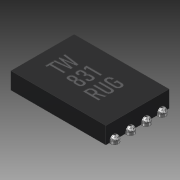
# Autodesk Inventor part: ATECC608A No Lead Crypto Auth
Saved by Autodesk Inventor 2016 (Build 200138000, 138)
## iProperties
Created: 2019-08-17
Part Number: ATECC608A No Lead Crypto Auth
Material: Generic
Document SubType Name: Modeling
Designer: Orest
Mass: 0.00326775 g
Surface Area: 0.184366 cm^2
Volume: 0.00326775 cm^3
Density: 1 g/cm^3
Appearance: Smooth - Black (BGA)
Catalog Web Link: http://ww1.microchip.com/downloads/en/DeviceDoc/40001977A.pdf
Author: Orest
Autodesk Inventor part; units mm, degrees
ref_plane "YZ Plane" through (0, 0, 0) normal (1, 0, 0) x (0, 1, 0)
ref_plane "XZ Plane" through (0, 0, 0) normal (0, 1, 0) x (-1, 0, 0)
sketch "Sketch10" plane through (0, 0, 0) normal (0, 1, 0) x (-1, 0, 0)
  line L0 (1, -1.5) -> (-1, -1.5)
  line L1 (-1, -1.5) -> (-1, 1.5)
  line L2 (-1, 1.5) -> (1, 1.5)
  line L3 (1, 1.5) -> (1, -1.5)
  point P0 (0, 0)
  point P1 (0, -1.5)
  point P2 (1, 0)
  dimension "d7" = 2
  dimension "d8" = 3
  constraints: 8 end point, 2 midpoint, 2 parallel, 1 horizontal, 1 horizontal alignment, 1 perpendicular, 1 vertical alignment
  measures "d7" distance of L1.end L2.end
  measures "d8" distance of L0.end L1.end
extrude "Extrusion4" add sketch "Sketch10" along normal blind 0.53
sketch "Sketch12" plane through (0, 0.53, 0) normal (0, 1, 0) x (1, 0, 0)
  line L0 (1, 1.5) -> (-1, 1.5) construction
  line L1 (-1, 1.5) -> (-1, -1.5) construction
  line L2 (-1, -1.5) -> (1, -1.5) construction
  line L3 (1, -1.5) -> (1, 1.5) construction
  line L4 (-1, 1.7) -> (1, 1.7) construction
  line L5 (1, 1.7) -> (1, -1.3) construction
  line L6 (1, -1.3) -> (-1, -1.3) construction
  line L7 (-1, -1.3) -> (-1, 1.7) construction
  line L8 (-1, 1.5) -> (-1, -1.5) projected
  line L9 (-0.2312, 1.0618) -> (-0.166, 1.0618)
  line L10 (-0.166, 1.0618) -> (-0.166, 0.6027)
  line L11 (-0.166, 0.6027) -> (-0.2312, 0.6027)
  line L12 (-0.2312, 0.6027) -> (-0.2312, 1.0618)
  line L13 (-0.32, 1.1027) -> (-0.0772, 1.1027)
  line L14 (-0.0772, 1.1027) -> (-0.0772, 1.0408)
  line L15 (-0.0772, 1.0408) -> (-0.32, 1.0408)
  line L16 (-0.32, 1.0408) -> (-0.32, 1.1027)
  line L17 (0.0974, 1.1027) -> (0.1449, 1.1027)
  line L18 (0.1449, 1.1027) -> (0.2077, 0.7166)
  line L19 (0.2077, 0.7166) -> (0.251, 1.1027)
  line L20 (0.251, 1.1027) -> (0.3163, 1.1027)
  line L21 (0.3163, 1.1027) -> (0.2473, 0.6027)
  line L22 (0.2473, 0.6027) -> (0.1763, 0.6027)
  line L23 (0.1763, 0.6027) -> (0.1235, 0.9421)
  line L24 (0.1235, 0.9421) -> (0.0661, 0.6027)
  line L25 (0.0661, 0.6027) -> (-0.005, 0.6027)
  line L26 (-0.005, 0.6027) -> (-0.0739, 1.1027)
  line L27 (-0.0739, 1.1027) -> (-0.0083, 1.1027)
  line L28 (-0.0083, 1.1027) -> (0.0351, 0.7166)
  line L29 (0.0351, 0.7166) -> (0.0974, 1.1027)
  spline S0 degree 2 poles (-0.2362, -0.0523) (-0.2713, -0.0523) (-0.3208, -0.0271) (-0.3468, 0.0216) (-0.3468, 0.0555) knots 0 0 0 1 2 3 3 3
  line L30 (-0.3468, 0.0555) -> (-0.3468, 0.136)
  spline S1 degree 2 poles (-0.3468, 0.136) (-0.3468, 0.1633) (-0.3192, 0.2066) (-0.294, 0.2186) knots 0 0 0 1 2 2 2
  spline S2 degree 2 poles (-0.294, 0.2186) (-0.3159, 0.2293) (-0.3398, 0.2648) (-0.3398, 0.2871) knots 0 0 0 1 2 2 2
  line L31 (-0.3398, 0.2871) -> (-0.3398, 0.354)
  spline S3 degree 2 poles (-0.3398, 0.354) (-0.3398, 0.3866) (-0.3154, 0.4337) (-0.2692, 0.4581) (-0.2362, 0.4581) knots 0 0 0 1 2 3 3 3
  spline S4 degree 2 poles (-0.2362, 0.4581) (-0.2027, 0.4581) (-0.1544, 0.4337) (-0.1292, 0.387) (-0.1292, 0.354) knots 0 0 0 1 2 3 3 3
  line L32 (-0.1292, 0.354) -> (-0.1292, 0.2871)
  spline S5 degree 2 poles (-0.1292, 0.2871) (-0.1292, 0.2648) (-0.154, 0.2285) (-0.1767, 0.2186) knots 0 0 0 1 2 2 2
  spline S6 degree 2 poles (-0.1767, 0.2186) (-0.1507, 0.2066) (-0.1226, 0.1633) (-0.1226, 0.136) knots 0 0 0 1 2 2 2
  line L33 (-0.1226, 0.136) -> (-0.1226, 0.0555)
  spline S7 degree 2 poles (-0.1226, 0.0555) (-0.1226, 0.0216) (-0.1495, -0.0271) (-0.2002, -0.0523) (-0.2362, -0.0523) knots 0 0 0 1 2 3 3 3
  spline S8 degree 2 poles (-0.2362, 0.0113) (-0.2213, 0.0113) (-0.199, 0.0225) (-0.1879, 0.0439) (-0.1879, 0.0588) knots 0 0 0 1 2 3 3 3
  line L34 (-0.1879, 0.0588) -> (-0.1879, 0.143)
  spline S9 degree 2 poles (-0.1879, 0.143) (-0.1879, 0.1562) (-0.199, 0.1752) (-0.2213, 0.1847) (-0.2362, 0.1847) knots 0 0 0 1 2 3 3 3
  spline S10 degree 2 poles (-0.2362, 0.1847) (-0.2506, 0.1847) (-0.2709, 0.1752) (-0.2816, 0.1562) (-0.2816, 0.143) knots 0 0 0 1 2 3 3 3
  line L35 (-0.2816, 0.143) -> (-0.2816, 0.058)
  spline S11 degree 2 poles (-0.2816, 0.058) (-0.2816, 0.0431) (-0.2709, 0.022) (-0.2506, 0.0113) (-0.2362, 0.0113) knots 0 0 0 1 2 3 3 3
  spline S12 degree 2 poles (-0.2362, 0.2467) (-0.2234, 0.2467) (-0.2044, 0.2574) (-0.1949, 0.2776) (-0.1949, 0.2921) knots 0 0 0 1 2 3 3 3
  line L36 (-0.1949, 0.2921) -> (-0.1949, 0.3457)
  spline S13 degree 2 poles (-0.1949, 0.3457) (-0.1949, 0.361) (-0.2044, 0.3829) (-0.2234, 0.3945) (-0.2362, 0.3945) knots 0 0 0 1 2 3 3 3
  spline S14 degree 2 poles (-0.2362, 0.3945) (-0.2486, 0.3945) (-0.2655, 0.3829) (-0.2746, 0.361) (-0.2746, 0.3453) knots 0 0 0 1 2 3 3 3
  line L37 (-0.2746, 0.3453) -> (-0.2746, 0.2917)
  spline S15 degree 2 poles (-0.2746, 0.2917) (-0.2746, 0.2772) (-0.2655, 0.257) (-0.2486, 0.2467) (-0.2362, 0.2467) knots 0 0 0 1 2 3 3 3
  spline S16 degree 2 poles (0.0467, -0.0523) (0.0099, -0.0523) (-0.0417, -0.0283) (-0.069, 0.0175) (-0.069, 0.0501) knots 0 0 0 1 2 3 3 3
  line L38 (-0.069, 0.0501) -> (-0.069, 0.0914)
  line L39 (-0.069, 0.0914) -> (-0.0033, 0.0914)
  line L40 (-0.0033, 0.0914) -> (-0.0033, 0.0547)
  spline S17 degree 2 poles (-0.0033, 0.0547) (-0.0033, 0.041) (0.0087, 0.0216) (0.031, 0.0113) (0.0467, 0.0113) knots 0 0 0 1 2 3 3 3
  spline S18 degree 2 poles (0.0467, 0.0113) (0.069, 0.0113) (0.0937, 0.0365) (0.0937, 0.0596) knots 0 0 0 1 2 2 2
  line L41 (0.0937, 0.0596) -> (0.0937, 0.129)
  spline S19 degree 2 poles (0.0937, 0.129) (0.0937, 0.1538) (0.0723, 0.1818) (0.0533, 0.1818) knots 0 0 0 1 2 2 2
  line L42 (0.0533, 0.1818) -> (0.0182, 0.1818)
  line L43 (0.0182, 0.1818) -> (0.0182, 0.2438)
  line L44 (0.0182, 0.2438) -> (0.0533, 0.2438)
  spline S20 degree 2 poles (0.0533, 0.2438) (0.0681, 0.2438) (0.0855, 0.2656) (0.0855, 0.2855) knots 0 0 0 1 2 2 2
  line L45 (0.0855, 0.2855) -> (0.0855, 0.3544)
  spline S21 degree 2 poles (0.0855, 0.3544) (0.0855, 0.3734) (0.0648, 0.3945) (0.0462, 0.3945) knots 0 0 0 1 2 2 2
  spline S22 degree 2 poles (0.0462, 0.3945) (0.033, 0.3945) (0.0145, 0.3846) (0.0045, 0.3668) (0.0045, 0.354) knots 0 0 0 1 2 3 3 3
  line L46 (0.0045, 0.354) -> (0.0045, 0.314)
  line L47 (0.0045, 0.314) -> (-0.0607, 0.314)
  line L48 (-0.0607, 0.314) -> (-0.0607, 0.3552)
  spline S23 degree 2 poles (-0.0607, 0.3552) (-0.0607, 0.3879) (-0.0351, 0.4337) (0.0145, 0.4581) (0.0495, 0.4581) knots 0 0 0 1 2 3 3 3
  spline S24 degree 2 poles (0.0495, 0.4581) (0.0979, 0.4581) (0.1507, 0.4044) (0.1507, 0.3552) knots 0 0 0 1 2 2 2
  line L49 (0.1507, 0.3552) -> (0.1507, 0.2851)
  spline S25 degree 2 poles (0.1507, 0.2851) (0.1507, 0.2669) (0.128, 0.2297) (0.1073, 0.2136) knots 0 0 0 1 2 2 2
  spline S26 degree 2 poles (0.1073, 0.2136) (0.1317, 0.2037) (0.159, 0.1591) (0.159, 0.129) knots 0 0 0 1 2 2 2
  line L50 (0.159, 0.129) -> (0.159, 0.058)
  spline S27 degree 2 poles (0.159, 0.058) (0.159, 0.0229) (0.1325, -0.0267) (0.0822, -0.0523) (0.0467, -0.0523) knots 0 0 0 1 2 3 3 3
  line L51 (0.3452, -0.0473) -> (0.2795, -0.0473)
  line L52 (0.2795, -0.0473) -> (0.2795, 0.385)
  line L53 (0.2795, 0.385) -> (0.2036, 0.3383)
  line L54 (0.2036, 0.3383) -> (0.2036, 0.406)
  line L55 (0.2036, 0.406) -> (0.2733, 0.4527)
  line L56 (0.2733, 0.4527) -> (0.3452, 0.4527)
  line L57 (0.3452, 0.4527) -> (0.3452, -0.0473)
  line L58 (-0.3947, -0.424) -> (-0.3022, -0.424)
  spline S28 degree 2 poles (-0.3022, -0.424) (-0.2849, -0.424) (-0.2597, -0.4108) (-0.2465, -0.386) (-0.2465, -0.3687) knots 0 0 0 1 2 3 3 3
  line L59 (-0.2465, -0.3687) -> (-0.2465, -0.3175)
  spline S29 degree 2 poles (-0.2465, -0.3175) (-0.2465, -0.2989) (-0.2597, -0.2725) (-0.2849, -0.2588) (-0.3022, -0.2588) knots 0 0 0 1 2 3 3 3
  line L60 (-0.3022, -0.2588) -> (-0.3947, -0.2588)
  line L61 (-0.3947, -0.2588) -> (-0.3947, -0.1969)
  line L62 (-0.3947, -0.1969) -> (-0.308, -0.1969)
  spline S30 degree 2 poles (-0.308, -0.1969) (-0.2684, -0.1969) (-0.2114, -0.2233) (-0.1813, -0.2745) (-0.1813, -0.3104) knots 0 0 0 1 2 3 3 3
  line L63 (-0.1813, -0.3104) -> (-0.1813, -0.3687)
  spline S31 degree 2 poles (-0.1813, -0.3687) (-0.1813, -0.4058) (-0.2114, -0.4583) (-0.2684, -0.4859) (-0.308, -0.4859) knots 0 0 0 1 2 3 3 3
  line L64 (-0.308, -0.4859) -> (-0.3947, -0.4859)
  line L65 (-0.3947, -0.4859) -> (-0.3947, -0.424)
  line L66 (-0.4253, -0.1969) -> (-0.3596, -0.1969)
  line L67 (-0.3596, -0.1969) -> (-0.3596, -0.6973)
  line L68 (-0.3596, -0.6973) -> (-0.4253, -0.6973)
  line L69 (-0.4253, -0.6973) -> (-0.4253, -0.1969)
  line L70 (-0.3084, -0.4702) -> (-0.2469, -0.4545)
  line L71 (-0.2469, -0.4545) -> (-0.1672, -0.6973)
  line L72 (-0.1672, -0.6973) -> (-0.2386, -0.6973)
  line L73 (-0.2386, -0.6973) -> (-0.3084, -0.4702)
  spline S32 degree 2 poles (0.0033, -0.7023) (-0.033, -0.7023) (-0.0842, -0.6754) (-0.1102, -0.6226) (-0.1102, -0.585) knots 0 0 0 1 2 3 3 3
  line L74 (-0.1102, -0.585) -> (-0.1102, -0.1973)
  line L75 (-0.1102, -0.1973) -> (-0.045, -0.1973)
  line L76 (-0.045, -0.1973) -> (-0.045, -0.5875)
  spline S33 degree 2 poles (-0.045, -0.5875) (-0.045, -0.6123) (-0.0202, -0.6387) (0.0033, -0.6387) knots 0 0 0 1 2 2 2
  spline S34 degree 2 poles (0.0033, -0.6387) (0.0268, -0.6387) (0.052, -0.6123) (0.052, -0.5875) knots 0 0 0 1 2 2 2
  line L77 (0.052, -0.5875) -> (0.052, -0.1973)
  line L78 (0.052, -0.1973) -> (0.1173, -0.1973)
  line L79 (0.1173, -0.1973) -> (0.1173, -0.585)
  spline S35 degree 2 poles (0.1173, -0.585) (0.1173, -0.6226) (0.0908, -0.6754) (0.04, -0.7023) (0.0033, -0.7023) knots 0 0 0 1 2 3 3 3
  line L80 (0.4253, -0.4281) -> (0.4253, -0.5743)
  spline S36 degree 2 poles (0.4253, -0.5743) (0.4253, -0.6147) (0.3968, -0.6721) (0.3431, -0.7023) (0.3051, -0.7023) knots 0 0 0 1 2 3 3 3
  spline S37 degree 2 poles (0.3051, -0.7023) (0.2667, -0.7023) (0.2114, -0.6738) (0.1829, -0.6197) (0.1829, -0.5813) knots 0 0 0 1 2 3 3 3
  line L81 (0.1829, -0.5813) -> (0.1829, -0.3204)
  spline S38 degree 2 poles (0.1829, -0.3204) (0.1829, -0.2799) (0.2114, -0.2225) (0.2651, -0.1919) (0.3031, -0.1919) knots 0 0 0 1 2 3 3 3
  spline S39 degree 2 poles (0.3031, -0.1919) (0.3402, -0.1919) (0.3931, -0.2213) (0.4211, -0.2774) (0.4211, -0.3166) knots 0 0 0 1 2 3 3 3
  line L82 (0.4211, -0.3166) -> (0.4211, -0.3414)
  line L83 (0.4211, -0.3414) -> (0.3514, -0.3414)
  line L84 (0.3514, -0.3414) -> (0.3514, -0.3166)
  spline S40 degree 2 poles (0.3514, -0.3166) (0.3514, -0.2972) (0.3402, -0.27) (0.3187, -0.2555) (0.3031, -0.2555) knots 0 0 0 1 2 3 3 3
  spline S41 degree 2 poles (0.3031, -0.2555) (0.2857, -0.2555) (0.2609, -0.2708) (0.2486, -0.2997) (0.2486, -0.3204) knots 0 0 0 1 2 3 3 3
  line L85 (0.2486, -0.3204) -> (0.2486, -0.5813)
  spline S42 degree 2 poles (0.2486, -0.5813) (0.2486, -0.5995) (0.2618, -0.6255) (0.2874, -0.6387) (0.3051, -0.6387) knots 0 0 0 1 2 3 3 3
  spline S43 degree 2 poles (0.3051, -0.6387) (0.3225, -0.6387) (0.3468, -0.6242) (0.3596, -0.5953) (0.3596, -0.5751) knots 0 0 0 1 2 3 3 3
  line L86 (0.3596, -0.5751) -> (0.3596, -0.49)
  line L87 (0.3596, -0.49) -> (0.3035, -0.49)
  line L88 (0.3035, -0.49) -> (0.3035, -0.4281)
  line L89 (0.3035, -0.4281) -> (0.4253, -0.4281)
  point P0 (0, 0)
  point P1 (0, 1.7)
  point P2 (0, 1.5)
  dimension "d32" = 0.2
  constraints: 2 equal length, 2 midpoint, 1 vertical alignment, 2 other
  measures "d32" distance between parallel lines of L2 L6
extrude "Extrusion6" cut sketch "Sketch12" against normal blind 0.01 contours L12 L15 L16 L13 L14 L10 L9 | L9 L10 L15 L12 | L15 L10 L11 L12 | L17 L18 L19 L20 L21 L22 L23 L24 L25 L26 L27 L28 L29 | S0 L30 S1 S2 L31 S3 S4 L32 S5 S6 L33 S7 | S16 L38 L39 L40 S17 S18 L41 S19 L42 L43 L44 S20 L45 S21 S22 L46 L47 L48 S23 S24 L49 S25 S26 L50 S27 | L51 L52 L53 L54 L55 L56 L57 | L65 L64 L67 L68 L69 L66 L61 L60 L58 | L58 L67 L64 L65 | L58 S28 L59 S29 L60 L67 L62 S30 L63 S31 L71 L70 L73 L64 | L60 L61 L62 L67 | L73 L70 L71 S31 | S31 L71 L72 L73 | S32 L74 L75 L76 S33 S34 L77 L78 L79 S35 | L80 S36 S37 L81 S38 S39 L82 L83 L84 S40 S41 L85 S42 S43 L86 L87 L88 L89
ref_plane "Work Plane1" through (0, -0.02, 0) normal (0, -1, 0) x (1, 0, 0)
sketch "Sketch11" plane through (0, -0.02, 0) normal (0, -1, 0) x (1, 0, 0)
  line L0 (-1, -1.5) -> (1, -1.5) construction
  line L1 (0.875, -1.65) -> (0.625, -1.65)
  line L2 (0.625, -1.65) -> (0.625, -1.05)
  line L3 (0.625, -1.05) -> (0.875, -1.05)
  line L4 (0.875, -1.05) -> (0.875, -1.65)
  line L5 (0.55, -0.6) -> (-0.55, -0.6)
  line L6 (-0.75, -0.4) -> (-0.75, 0.4)
  line L7 (-0.55, 0.6) -> (0.55, 0.6)
  line L8 (0.75, 0.4) -> (0.75, -0.4)
  line L9 (0.375, -1.65) -> (0.125, -1.65)
  line L10 (0.125, -1.65) -> (0.125, -1.05)
  line L11 (0.125, -1.05) -> (0.375, -1.05)
  line L12 (0.375, -1.05) -> (0.375, -1.65)
  line L13 (-0.125, -1.65) -> (-0.375, -1.65)
  line L14 (-0.375, -1.65) -> (-0.375, -1.05)
  line L15 (-0.375, -1.05) -> (-0.125, -1.05)
  line L16 (-0.125, -1.05) -> (-0.125, -1.65)
  line L17 (-0.625, -1.65) -> (-0.875, -1.65)
  line L18 (-0.875, -1.65) -> (-0.875, -1.05)
  line L19 (-0.875, -1.05) -> (-0.625, -1.05)
  line L20 (-0.625, -1.05) -> (-0.625, -1.65)
  line L21 (0, -1.5) -> (0, 1.5) construction
  line L22 (1, 0) -> (-1, 0) construction
  line L23 (0.875, 1.65) -> (0.625, 1.65)
  line L24 (0.625, 1.65) -> (0.625, 1.05)
  line L25 (0.625, 1.05) -> (0.875, 1.05)
  line L26 (0.875, 1.05) -> (0.875, 1.65)
  line L27 (0.375, 1.65) -> (0.125, 1.65)
  line L28 (0.125, 1.65) -> (0.125, 1.05)
  line L29 (0.125, 1.05) -> (0.375, 1.05)
  line L30 (0.375, 1.05) -> (0.375, 1.65)
  line L31 (-0.125, 1.65) -> (-0.375, 1.65)
  line L32 (-0.375, 1.65) -> (-0.375, 1.05)
  line L33 (-0.375, 1.05) -> (-0.125, 1.05)
  line L34 (-0.125, 1.05) -> (-0.125, 1.65)
  line L35 (-0.625, 1.65) -> (-0.875, 1.65)
  line L36 (-0.875, 1.65) -> (-0.875, 1.05)
  line L37 (-0.875, 1.05) -> (-0.625, 1.05)
  line L38 (-0.625, 1.05) -> (-0.625, 1.65)
  arc A0 (0.55, -0.6) -> (0.75, -0.4) centre (0.55, -0.4) ccw
  arc A1 (-0.75, -0.4) -> (-0.55, -0.6) centre (-0.55, -0.4) ccw
  arc A2 (-0.55, 0.6) -> (-0.75, 0.4) centre (-0.55, 0.4) ccw
  arc A3 (0.75, 0.4) -> (0.55, 0.6) centre (0.55, 0.4) ccw
  line L39 (-1, -1.5) -> (1, -1.5) projected
  line L40 (1, -1.5) -> (1, 1.5) projected
  line L41 (1, 1.5) -> (-1, 1.5) projected
  line L42 (-1, 1.5) -> (-1, -1.5) projected
  line L43 (1, -1.5) -> (1, 1.5) projected
  point P0 (0.75, -0.6)
  point P1 (-0.75, -0.6)
  point P2 (0, -0.6)
  point P3 (-0.75, 0)
  dimension "d12" = 0.25
  dimension "d16" = 0.5
  dimension "d21" = 0.15
  dimension "d22" = 0.45
  dimension "d23" = 1.5
  dimension "d24" = 1.2
  dimension "d25" = 0.45
  dimension "d27" = 0.2
  constraints: 78 end point, 16 symmetric about line, 9 midpoint, 8 point on circle, 8 tangent, 6 point on line, 5 parallel, 4 centre point, 3 equal radius, 3 horizontal, 2 perpendicular, 25 other
  measures "d12" distance between parallel lines of L4 L2
  measures "d16" distance of L1.start L9.start
  measures "d21" distance between parallel lines of L17 L0
  measures "d22" distance between parallel lines of L0 L19
  measures "d23" distance of point (0.75, -0.6) point (-0.75, -0.6)
  measures "d24" distance between parallel lines of L7 L5
  measures "d25" distance between parallel lines of L19 L5
  measures "d27" radius of A0
extrude "Extrusion5" add sketch "Sketch11" against normal blind 0.2 contours L1 L2 L39 L4 | L39 L2 L3 L4 | L39 L10 L11 L12 | L12 L9 L10 L39 | L41 L24 L23 L26 | L26 L25 L24 L41 | L39 L14 L15 L16 | L16 L13 L14 L39 | L41 L28 L27 L30 | L30 L29 L28 L41 | L39 L18 L19 L20 | L20 L17 L18 L39 | L41 L32 L31 L34 | L34 L33 L32 L41 | L41 L36 L35 L38 | L38 L37 L36 L41 | L5 A1 L6 A2 L7 A3 L8 A0
fillet "Fillet1" radius 0.125 40 edges at (-0.875, 0.18, -1.575) (-0.75, 0.18, -1.65) (-0.625, 0.18, -1.575) (-0.625, 0.08, -1.65) (-0.875, 0.08, -1.65) (-0.375, 0.08, -1.65) (-0.25, 0.18, -1.65) (-0.375, 0.18, -1.575) (-0.125, 0.18, -1.575) (-0.125, 0.08, -1.65) (0.125, 0.08, -1.65) (0.125, 0.18, -1.575) (0.375, 0.08, -1.65) (0.375, 0.18, -1.575) (0.25, 0.18, -1.65) (0.75, 0.18, -1.65) (0.625, 0.08, -1.65) (0.875, 0.08, -1.65) (0.875, 0.18, -1.575) (0.625, 0.18, -1.575) (-0.75, 0.18, 1.65) (-0.25, 0.18, 1.65) (0.25, 0.18, 1.65) (0.75, 0.18, 1.65) (0.875, 0.08, 1.65) (0.625, 0.08, 1.65) (0.375, 0.08, 1.65) (0.125, 0.08, 1.65) (0.125, 0.18, 1.575) (0.375, 0.18, 1.575) (0.625, 0.18, 1.575) (0.875, 0.18, 1.575) (-0.125, 0.18, 1.575) (-0.625, 0.18, 1.575) (-0.875, 0.18, 1.575) (-0.875, 0.08, 1.65) (-0.625, 0.08, 1.65) (-0.375, 0.08, 1.65) (-0.125, 0.08, 1.65) (-0.375, 0.18, 1.575)
body "Solid4"
